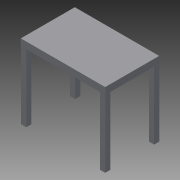
# Autodesk Inventor part: tables
Saved by Autodesk Inventor 2015 (Build 190159000, 159)
## iProperties
Created: 2014-10-26
Part Number: tables
Material: Generic
Document SubType Name: Modeling
Designer: ericd_000
Density: 1 g/cm^3
Appearance: Default
Author: ericd_000
Autodesk Inventor part; units mm, degrees
ref_plane "YZ Plane" through (0, 0, 0) normal (1, 0, 0) x (0, 1, 0)
ref_plane "XZ Plane" through (0, 0, 0) normal (0, 1, 0) x (-1, 0, 0)
ref_plane "XY Plane" through (0, 0, 0) normal (0, 0, 1) x (1, 0, 0)
sketch "Sketch1" plane through (0, 0, 0) normal (0, 0, 1) x (1, 0, 0)
  line L0 (-625, 400) -> (625, 400)
  line L1 (625, 400) -> (625, -400)
  line L2 (625, -400) -> (-625, -400)
  line L3 (-625, -400) -> (-625, 400)
  point P0 (0, 0)
  point P1 (-625, 0)
  point P2 (0, 400)
  dimension "d0" = 1250
  dimension "d1" = 800
  constraints: 8 end point, 2 midpoint, 2 parallel, 1 horizontal, 1 horizontal alignment, 1 perpendicular, 1 vertical alignment
  measures "d0" distance of L0.start L0.end
  measures "d1" distance of L2.end L0.start
extrude "Extrusion1" add sketch "Sketch1" along normal blind 100
sketch "Sketch2" plane through (0, 0, 0) normal (0, 0, -1) x (-1, 0, 0)
  line L0 (-625, 400) -> (-550, 400)
  line L1 (-550, 400) -> (-550, 325)
  line L2 (-550, 325) -> (-625, 325)
  line L3 (-625, 325) -> (-625, 400)
  line L4 (545, 400) -> (620, 400)
  line L5 (620, 400) -> (620, 325)
  line L6 (620, 325) -> (545, 325)
  line L7 (545, 325) -> (545, 400)
  line L8 (-625, -325) -> (-550, -325)
  line L9 (-550, -325) -> (-550, -400)
  line L10 (-550, -400) -> (-625, -400)
  line L11 (-625, -400) -> (-625, -325)
  line L12 (545, -325) -> (620, -325)
  line L13 (620, -325) -> (620, -400)
  line L14 (620, -400) -> (545, -400)
  line L15 (545, -400) -> (545, -325)
  point P0 (0, 0)
  dimension "d4" = 75
  dimension "d5" = 75
  dimension "d8" = 1170
  dimension "d11" = 725
  constraints: 32 end point, 2 collinear, 2 horizontal, 2 parallel, 1 perpendicular, 1 vertical, 22 other
  measures "d4" distance of L0.end L1.end
  measures "d5" distance of L1.end L2.end
  measures "d8" distance of L2.end L7.start
  measures "d11" distance of L2.end L11.start
extrude "Extrusion2" add sketch "Sketch2" along normal blind 1000
body "Solid1"
